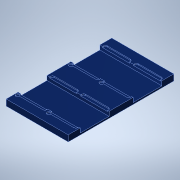
# Autodesk Inventor part: Assembly Plate
Saved by Autodesk Inventor 2022 (Build 260153000, 153)
## iProperties
Created: 2021-01-11
Part Number: Assembly Plate
Material: Aluminum, Anodized Blue
Document SubType Name: Modeling
Designer: caleb
Density: 2.7 g/cm^3
Appearance: Anodized - Blue
Author: caleb
Autodesk Inventor part; units mm, degrees
ref_plane "YZ Plane" through (0, 0, 0) normal (1, 0, 0) x (0, 1, 0)
ref_plane "XZ Plane" through (0, 0, 0) normal (0, 1, 0) x (-1, 0, 0)
ref_plane "XY Plane" through (0, 0, 0) normal (0, 0, 1) x (1, 0, 0)
sketch "Sketch1" plane through (0, 0, 0) normal (0, 1, 0) x (-1, 0, 0)
  line L0 (-63.5, 107.95) -> (63.5, 107.95)
  line L1 (63.5, 107.95) -> (63.5, -107.95)
  line L2 (63.5, -107.95) -> (-63.5, -107.95)
  line L3 (-63.5, -107.95) -> (-63.5, 107.95)
  line L4 (-63.5, 107.95) -> (63.5, -107.95) construction
  line L5 (63.5, 107.95) -> (-63.5, -107.95) construction
  point P0 (0, 0)
  dimension "d0" = 127
  dimension "d1" = 215.9
  constraints: 12 end point, 2 midpoint, 2 parallel, 1 horizontal, 1 perpendicular
  measures "d0" distance of L1.end L2.end
  measures "d1" distance of L0.end L1.end
extrude "Extrusion1" add sketch "Sketch1" along normal blind 12.7
sketch "Sketch13" plane through (0, 12.7, 0) normal (0, 1, 0) x (1, 0, 0)
  line L0 (-54, -18.475) -> (-7, -18.475)
  line L1 (-3, -22.475) -> (-3, -85.475)
  line L2 (-7, -89.475) -> (-58, -89.475)
  line L3 (-58, -89.475) -> (-58, -22.475)
  line L4 (-58, -18.475) -> (-3, -89.475) construction
  line L5 (-3, -18.475) -> (-58, -89.475) construction
  line L6 (-63.5, -107.95) -> (63.5, -107.95) projected
  line L7 (-63.5, 107.95) -> (-63.5, -107.95) projected
  arc A0 (-54, -18.475) -> (-58, -22.475) centre (-54, -22.475) ccw
  arc A1 (-3, -22.475) -> (-7, -18.475) centre (-7, -22.475) ccw
  arc A2 (-7, -89.475) -> (-3, -85.475) centre (-7, -85.475) ccw
  circle A3 centre (-58, -89.475) radius 4
  arc A4 (9.5, -18.475) -> (5.5, -22.475) centre (9.5, -22.475) ccw
  line L8 (9.5, -18.475) -> (56.5, -18.475)
  line L9 (5.5, -89.475) -> (5.5, -22.475)
  circle A5 centre (5.5, -89.475) radius 4
  line L10 (60.5, -22.475) -> (60.5, -85.475)
  line L11 (56.5, -89.475) -> (5.5, -89.475)
  line L12 (5.5, -18.475) -> (60.5, -89.475) construction
  line L13 (60.5, -18.475) -> (5.5, -89.475) construction
  arc A6 (56.5, -89.475) -> (60.5, -85.475) centre (56.5, -85.475) ccw
  arc A7 (60.5, -22.475) -> (56.5, -18.475) centre (56.5, -22.475) ccw
  arc A8 (-54, 89.475) -> (-58, 85.475) centre (-54, 85.475) ccw
  line L14 (-54, 89.475) -> (-7, 89.475)
  line L15 (-58, 18.475) -> (-58, 85.475)
  circle A9 centre (-58, 18.475) radius 4
  line L16 (-3, 85.475) -> (-3, 22.475)
  line L17 (-7, 18.475) -> (-58, 18.475)
  line L18 (-58, 89.475) -> (-3, 18.475) construction
  line L19 (-3, 89.475) -> (-58, 18.475) construction
  arc A10 (-7, 18.475) -> (-3, 22.475) centre (-7, 22.475) ccw
  arc A11 (-3, 85.475) -> (-7, 89.475) centre (-7, 85.475) ccw
  arc A12 (9.5, 89.475) -> (5.5, 85.475) centre (9.5, 85.475) ccw
  line L20 (9.5, 89.475) -> (56.5, 89.475)
  line L21 (5.5, 18.475) -> (5.5, 85.475)
  circle A13 centre (5.5, 18.475) radius 4
  line L22 (60.5, 85.475) -> (60.5, 22.475)
  line L23 (56.5, 18.475) -> (5.5, 18.475)
  line L24 (5.5, 89.475) -> (60.5, 18.475) construction
  line L25 (60.5, 89.475) -> (5.5, 18.475) construction
  arc A14 (56.5, 18.475) -> (60.5, 22.475) centre (56.5, 22.475) ccw
  arc A15 (60.5, 85.475) -> (56.5, 89.475) centre (56.5, 85.475) ccw
  point P0 (0, 0)
  point P1 (-30.5, -53.975)
  point P2 (63.5, 0)
  point P3 (33, -53.975)
  point P4 (0, 107.95)
  point P5 (-30.5, 53.975)
  point P6 (63.5, 107.95)
  point P7 (33, 53.975)
  point P8 (-58, 22.475)
  point P9 (-54, 18.475)
  point P10 (5.5, 22.475)
  point P11 (9.5, 18.475)
  point P12 (5.5, -85.475)
  point P13 (9.5, -89.475)
  point P14 (-58, -85.475)
  point P15 (-54, -89.475)
  dimension "d142" = 71
  dimension "d143" = 55
  dimension "d146" = 33
  dimension "d147" = 30.5
  dimension "d148" = 53.975
  dimension "d149" = 53.975
  dimension "d150" = 4
  dimension "d151" = 8
  dimension "d154" = 63.5
  dimension "d157" = 107.95
  constraints: 48 end point, 24 point on circle, 24 point on line, 16 centre point, 8 midpoint, 6 tangent, 4 coincident, 2 equal radius, 2 horizontal, 2 parallel, 1 perpendicular, 1 vertical, 78 other
  measures "d142" distance of L2.end L4.start
  measures "d143" distance of L4.start L5.start
  measures "d146" distance from line of L7 point (-30.5, -53.975)
  measures "d147" horizontal distance of point (0, 0) point (-30.5, -53.975)
  measures "d148" vertical distance of point (0, 0) point (-30.5, -53.975)
  measures "d149" distance from line of L6 point (-30.5, -53.975)
  measures "d150" radius of A0
  measures "d151" diameter of A3
  measures "d154" distance of L4.start L12.start
  measures "d157" distance of L4.start L18.start
extrude "Extrusion12" cut sketch "Sketch13" against normal blind 2
sketch "Sketch15" plane through (0, 12.7, 0) normal (0, 1, 0) x (1, 0, 0)
  line L0 (63.5, 107.95) -> (63.5, -107.95) projected
  line L1 (-63.5, 83.475) -> (63.5, 83.475)
  line L2 (63.5, 83.475) -> (63.5, 24.475)
  line L3 (63.5, 24.475) -> (-63.5, 24.475)
  line L4 (-63.5, 24.475) -> (-63.5, 83.475)
  line L5 (-63.5, 83.475) -> (63.5, 24.475) construction
  line L6 (63.5, 83.475) -> (-63.5, 24.475) construction
  line L7 (63.5, 107.95) -> (-63.5, 107.95) projected
  line L8 (-63.5, -24.475) -> (63.5, -24.475)
  line L9 (63.5, -24.475) -> (63.5, -83.475)
  line L10 (63.5, -83.475) -> (-63.5, -83.475)
  line L11 (-63.5, -83.475) -> (-63.5, -24.475)
  line L12 (-63.5, -24.475) -> (63.5, -83.475) construction
  line L13 (63.5, -24.475) -> (-63.5, -83.475) construction
  point P0 (0, 0)
  point P1 (0, 53.975)
  point P2 (63.5, 83.475)
  point P3 (0, 53.975)
  point P4 (0, -53.975)
  point P5 (0, -53.975)
  point P6 (63.5, -24.475)
  dimension "d171" = 59
  dimension "d172" = 24.475
  dimension "d173" = 24.475
  dimension "d178" = 107.95
  constraints: 24 end point, 5 midpoint, 2 parallel, 1 horizontal, 1 perpendicular, 1 point on line, 1 vertical, 1 vertical alignment, 12 other
  measures "d171" distance between parallel lines of L3 L1
  measures "d172" distance between parallel lines of L7 L1
  measures "d173" distance from line of point (0, 0) L3
  measures "d178" distance of L1.start L8.start
extrude "Extrusion14" cut sketch "Sketch15" against normal blind 9
body "Solid1"
